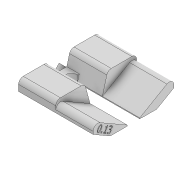
# Autodesk Inventor part: alex_clip
Saved by Autodesk Inventor 2022 (Build 260153000, 153)
## iProperties
Created: 2022-08-18
Part Number: alex_clip
Material: Generic
Document SubType Name: Modeling
Designer: dsdan
Density: 1 g/cm^3
Appearance: Default
Author: dsdan
Autodesk Inventor part; units mm, degrees
ref_plane "YZ Plane" through (0, 0, 0) normal (1, 0, 0) x (0, 1, 0)
ref_plane "XZ Plane" through (0, 0, 0) normal (0, 1, 0) x (-1, 0, 0)
ref_plane "XY Plane" through (0, 0, 0) normal (0, 0, 1) x (1, 0, 0)
sketch "Sketch1" plane through (0, 0, 0) normal (1, 0, 0) x (0, 1, 0)
  arc A0 (3.8, 2.5025) -> (-1, 4.4387) centre (0, 0) ccw
  line L0 (3.8, 2.5025) -> (3.8, -2.5025)
  line L1 (-1, 4.4387) -> (-1, -4.4387)
  arc A1 (3.8, -2.5025) -> (3.8, 2.5025) centre (0, 0) ccw construction
  arc A2 (-1, 4.4387) -> (-1, -4.4387) centre (0, 0) ccw construction
  arc A3 (-1, -4.4387) -> (3.8, -2.5025) centre (0, 0) ccw
  dimension "d0" = 9.1
  dimension "d5" = 4.8
  dimension "d40" = 3.8
  constraints: 9 point on circle, 4 centre point, 4 end point, 1 coincident, 1 vertical
  measures "d0" diameter of A0
  measures "d5" distance between parallel lines of L1 L0
  measures "d40" distance from line of point (0, 0) L0
extrude "Extrusion1" add sketch "Sketch1" along normal blind 28
sketch "Sketch9" plane through (28, 0, 0) normal (1, 0, 0) x (0, 0, -1)
  arc A0 (-2.5025, 3.8) -> (-4.4387, -1) centre (0, 0) ccw projected
  line L0 (-4.1788, 1.8) -> (4.1788, 1.8)
  arc A1 (4.4387, -1) -> (2.5025, 3.8) centre (0, 0) ccw projected
  line L1 (2.5025, 3.8) -> (-2.5025, 3.8) projected
  line L2 (-4.2305, 1.675) -> (4.2305, 1.675) construction
  dimension "d69" = 2.125
  dimension "d70" = 0.125
  constraints: 4 end point, 4 point on circle, 2 horizontal
  measures "d69" distance between parallel lines of L2 L1
  measures "d70" distance between parallel lines of L2 L0
extrude "Extrusion9" cut sketch "Sketch9" against normal blind 24
sketch "Sketch3" plane through (0, 3.8, 2.5025) normal (0, 1, 0) x (1, 0, 0)
  circle A0 centre (8, 2.5025) radius 2
  line L0 (8, 4.5025) -> (28, 4.5025)
  line L1 (8, 0.5025) -> (28, 0.5025)
  line L2 (28, 5.005) -> (28, 0) projected
  line L3 (0, 5.005) -> (0, 0) projected
  point P0 (0, 2.5025)
  dimension "d10" = 4
  dimension "d61" = 8
  constraints: 4 end point, 2 horizontal, 2 point on circle, 2 point on line, 2 tangent, 1 centre point, 1 horizontal alignment
  measures "d10" diameter of A0
  measures "d61" distance from line of L3 A0.centre
extrude "Extrusion3" cut sketch "Sketch3" against normal through all
sketch "Sketch6" plane through (28, 0, 0) normal (1, 0, 0) x (0, 0, -1)
  line L0 (-2, 1.8) -> (-2, -1) projected
  circle A0 centre (0, 0) radius 3.05
  line L1 (-2.6268, 1.55) -> (2.6268, 1.55)
  line L2 (-2.6268, -1.55) -> (2.6268, -1.55)
  dimension "d42" = 6.1
  dimension "d43" = 3.1
  dimension "d44" = 1.55
  constraints: 4 end point, 4 point on circle, 1 centre point, 1 coincident, 1 horizontal
  measures "d42" diameter of A0
  measures "d43" distance between parallel lines of L1 L2
  measures "d44" distance from line of point (0, 0) L1
extrude "Extrusion7" cut sketch "Sketch6" against normal through all contours A0 L2 L1
fillet "Fillet3" radius 0.3 2 edges at (14, 1.55, 2.6268) (14, 1.55, -2.6268)
sketch "Sketch7" plane through (8, 3.8, -2) normal (0, 0, 1) x (1, 0, 0)
  circle A0 centre (1, -3.8) radius 1.5
  line L0 (1, -5.3) -> (20, -5.3)
  line L1 (20, -5.3) -> (20, -2.3)
  line L2 (1, -2.3) -> (20, -2.3)
  line L3 (20, -4.8) -> (0, -4.8) projected
  line L4 (20, -2) -> (20, -2.25) projected
  line L5 (-8, -4.8) -> (-8, 0) projected
  dimension "d28" = 3
  dimension "d33" = 2.5
  dimension "d60" = 9
  constraints: 6 end point, 2 perpendicular, 2 point on circle, 2 tangent, 1 centre point, 1 collinear, 1 horizontal
  measures "d28" diameter of A0
  measures "d33" distance between parallel lines of L3 L2
  measures "d60" distance from line of L5 A0.centre
extrude "Extrusion6" cut sketch "Sketch7" along normal through all both and the other way through all
sketch "Sketch12" plane through (0, 0, 0) normal (-1, 0, 0) x (0, 0, 1)
  line L0 (-4.55, -1) -> (4.55, -1) construction
  line L1 (4.55, -1) -> (4.55, 2.5)
  line L2 (4.55, 2.5) -> (-4.55, 2.5) construction
  line L3 (-4.55, 2.5) -> (-4.55, -1)
  arc A0 (-2.5025, 3.8) -> (-4.4387, -1) centre (0, 0) ccw projected
  arc A1 (4.4387, -1) -> (2.5025, 3.8) centre (0, 0) ccw projected
  line L4 (-2.8814, -1) -> (-4.4387, -1) projected
  line L5 (-4.55, 2.5) -> (-2.05, 0)
  line L6 (-4.55, 2.5) -> (-1.0145, 2.5) construction
  line L7 (-2.05, 0) -> (2.05, 0)
  line L8 (2.05, 0) -> (4.55, 2.5)
  line L9 (-4.55, 2.5) -> (-4.55, 4.4728)
  line L10 (-4.55, 4.4728) -> (4.55, 4.4728)
  line L11 (4.55, 4.4728) -> (4.55, 2.5)
  dimension "d57" = 3.5
  dimension "d58" = 45
  dimension "d59" = 45
  constraints: 22 end point, 3 horizontal, 3 perpendicular, 2 parallel, 2 tangent, 1 collinear, 1 equal length, 1 vertical
  measures "d57" distance between parallel lines of L0 L2
  measures "d58" angle of L5 L6
  measures "d59" angle of L2 L8
extrude "Extrusion11" cut sketch "Sketch12" against normal blind 4 contours L8 L7 L5 L9 L10 L11
sketch "Sketch4" plane through (28, 0, 0) normal (1, 0, 0) x (0, 0, -1)
  arc A0 (-4.1788, 1.8) -> (-4.2956, 1.5) centre (0, 0) ccw projected
  line L0 (-2, 1.8) -> (-13, 8.1509)
  line L1 (-2, 1.8) -> (10.7017, 1.8) construction
  line L2 (-13, 8.1509) -> (-13, 1.5)
  line L3 (2.6153, 1.5) -> (4.2956, 1.5) projected
  line L4 (-4.2956, 1.5) -> (4.2956, 1.5) projected
  line L5 (-13, 1.5) -> (-4.2956, 1.5)
  arc A1 (4.2956, 1.5) -> (4.1788, 1.8) centre (0, 0) ccw projected
  line L6 (2, 1.8) -> (2, 1.55) projected
  line L7 (-4.2956, 1.5) -> (-2.6153, 1.5) projected
  line L8 (-2.4495, 1.55) -> (-2, 1.55) projected
  arc A2 (2.6153, 1.5) -> (2.4495, 1.55) centre (2.4495, 1.25) ccw projected
  line L9 (4.1788, 1.8) -> (2, 1.8) projected
  arc A3 (-2.4495, 1.55) -> (-2.6153, 1.5) centre (-2.4495, 1.25) ccw projected
  line L10 (-2, 1.55) -> (-2, 1.8) projected
  line L11 (-2, 1.8) -> (-4.1788, 1.8) projected
  line L12 (2, 1.55) -> (2.4495, 1.55) projected
  point P0 (-4.4387, -1)
  point P1 (-1.5, 2.3)
  dimension "d16" = 30
  dimension "d21" = 11
  constraints: 8 end point, 1 collinear, 1 equal length, 1 horizontal, 1 perpendicular
  measures "d16" angle of L1 L0
  measures "d21" distance from line of L0.start L2
extrude "Extrusion4" add sketch "Sketch4" against normal blind 12 contours A0 L5 L2 L0 L11
sketch "Sketch5" plane through (16, 0, 0) normal (-1, 0, 0) x (0, 0, 1)
  line L0 (-2, 1.8) -> (-2, 1.55) projected
  arc A0 (-4.1788, 1.8) -> (-4.2956, 1.5) centre (0, 0) ccw projected
  line L1 (-2, 1.8) -> (-3.7017, 8.1509)
  line L2 (-3.7017, 8.1509) -> (-13, 8.1509)
  line L3 (-13, 8.1509) -> (-13, 1.5)
  line L4 (13, 1.5) -> (2.6153, 1.5) projected
  arc A1 (-4.1788, 1.8) -> (-4.2956, 1.5) centre (0, 0) ccw projected
  line L5 (-13, 1.5) -> (-4.2956, 1.5)
  line L6 (-2.6153, 1.5) -> (-4.2956, 1.5) projected
  line L7 (-2, 1.55) -> (-2.4495, 1.55) projected
  arc A2 (-2.4495, 1.55) -> (-2.6153, 1.5) centre (-2.4495, 1.25) ccw projected
  line L8 (-4.1788, 1.8) -> (-2, 1.8) projected
  arc A3 (2.6153, 1.5) -> (2.4495, 1.55) centre (2.4495, 1.25) ccw projected
  line L9 (2.4495, 1.55) -> (2, 1.55) projected
  line L10 (2, 1.55) -> (2, 1.8) projected
  line L11 (2, 1.8) -> (13, 8.1509) projected
  line L12 (13, 8.1509) -> (13, 1.5) projected
  dimension "d25" = 11
  dimension "d49" = 75
  constraints: 8 end point, 2 horizontal, 1 perpendicular, 1 point on line
  measures "d25" distance between parallel lines of L3 L0
  measures "d49" angle of L8 L1
extrude "Extrusion5" add sketch "Sketch5" along normal blind 12 contours L8 A0 L5 L3 L2 L1
fillet "Fillet1" radius 1.5 3 edges at (22, 8.1509, 13) (10, 8.1509, -13) (10, 8.1509, -3.7017)
mirror "Mirror1" about plane through (0, 0, 0) normal (0, 0, 1) of "Extrusion5", "Extrusion4", "Fillet1"
sketch "Sketch8" plane through (28, 0, 0) normal (1, 0, 0) x (0, 0, -1)
  line L0 (13, 1.5) -> (2.6153, 1.5) projected
  line L1 (-2.6153, 1.5) -> (-4.2956, 1.5) projected
  line L2 (-13, 5.5528) -> (-13, 1.5) projected
  line L3 (-2, 1.8) -> (-10.75, 6.8518) construction
  line L4 (2, 1.8) -> (2, 1.55) projected
  line L5 (2, 1.55) -> (2.4495, 1.55) projected
  arc A0 (2.6153, 1.5) -> (2.4495, 1.55) centre (2.4495, 1.25) ccw projected
  line L6 (-13, 1.5) -> (-2.6153, 1.5) projected
  arc A1 (-10.75, 6.8518) -> (-13, 5.5528) centre (-11.5, 5.5528) ccw projected
  line L7 (-13, 4.6868) -> (-7.4804, 1.5)
  arc A2 (-2.4495, 1.55) -> (-2.6153, 1.5) centre (-2.4495, 1.25) ccw projected
  line L8 (-2.4495, 1.55) -> (-2, 1.55) projected
  line L9 (-2, 1.55) -> (-2, 1.8) projected
  line L10 (13, 5.5528) -> (13, 1.5) projected
  arc A3 (13, 5.5528) -> (10.75, 6.8518) centre (11.5, 5.5528) ccw projected
  line L11 (2, 1.8) -> (10.75, 6.8518) projected
  arc A4 (-10.75, 6.8518) -> (-13, 5.5528) centre (-11.5, 5.5528) ccw projected
  line L12 (-13, 5.5528) -> (-13, 1.5) projected
  line L13 (-2, 1.8) -> (-10.75, 6.8518) construction
  point P0 (0, 0)
  point P1 (-10.5, 7.4962)
  point P2 (-13, 4.6868)
  dimension "d68" = 3
  constraints: 2 end point, 1 parallel, 1 point on line, 1 other
  measures "d68" distance between parallel lines of L3 L7
extrude "Extrusion8" cut sketch "Sketch8" against normal through all contours L7 L6 L2
mirror "Mirror2" about plane through (0, 0, 0) normal (0, 0, 1) of "Extrusion8"
sketch "Sketch11" plane through (0, 3.8, 2.5025) normal (0, 1, 0) x (1, 0, 0)
  arc A0 (8, 4.5025) -> (8, 0.5025) centre (8, 2.5025) ccw projected
  arc A1 (8, 4.5025) -> (8, 0.5025) centre (8, 2.5025) ccw projected
  line L0 (4, 0.5025) -> (4, -0.4975)
  line L1 (4, -0.4975) -> (8, -0.4975)
  line L2 (8, -0.4975) -> (8, 0.5025)
  line L3 (8, 4.5025) -> (4, 4.5025) construction
  line L4 (4, 4.5025) -> (4, 5.5025)
  line L5 (4, 5.5025) -> (8, 5.5025)
  line L6 (8, 5.5025) -> (8, 4.5025)
  line L7 (4, 4.5025) -> (4, 0.5025) projected
  line L8 (8, 4.5025) -> (4, 4.5025) projected
  line L9 (4, 0.5025) -> (8, 0.5025) construction
  point P0 (7.5077, 4.441)
  constraints: 12 end point, 2 collinear, 2 parallel
extrude "Extrusion10" add sketch "Sketch11" against normal up to surface (2 mm away)
sketch "Sketch13" plane through (4, 1.6589, -7.7555) normal (0, -0.8660254, -0.5) x (0, 0.5, -0.8660254)
  line L0 (-0.3177, 24) -> (6.0558, 24) construction
  line L1 (6.0558, 24) -> (6.0558, 12) construction
  line L2 (6.0558, 12) -> (-0.3177, 12) construction
  line L3 (-0.3177, 12) -> (-0.3177, 24) construction
  line L4 (6.0558, 24) -> (6.0558, 0) projected
  line L5 (-0.3177, 12) -> (6.0558, 12) construction
  line L6 (6.0558, 12) -> (6.0558, 0) construction
  line L7 (6.0558, 0) -> (-0.3177, 0) construction
  line L8 (-0.3177, 0) -> (-0.3177, 12) construction
  line L9 (-0.3177, 0) -> (-0.3177, 24) projected
  line L10 (7.0378, 12) -> (6.4888, 12) projected
  line L11 (7.0378, 0) -> (6.0558, 0) projected
  line L12 (-0.3177, 24) -> (6.0558, 24) projected
  spline S0 degree 2 poles (1.0114, 21.0934) (0.9187, 21.0934) (0.7355, 21.0482) (0.647, 21.0132) knots 0 0 0 1 2 2 2
  spline S1 degree 2 poles (0.647, 21.0132) (0.5647, 20.9782) (0.4433, 20.9041) (0.3959, 20.8711) knots 0 0 0 1 2 2 2
  line L13 (0.3959, 20.8711) -> (0.3753, 20.8711)
  line L14 (0.3753, 20.8711) -> (0.3753, 21.2313)
  spline S2 degree 2 poles (0.3753, 21.2313) (0.4865, 21.291) (0.8673, 21.3878) (1.0381, 21.3878) knots 0 0 0 1 2 2 2
  spline S3 degree 2 poles (1.0381, 21.3878) (1.211, 21.3878) (1.4683, 21.3178) (1.5733, 21.2437) knots 0 0 0 1 2 2 2
  spline S4 degree 2 poles (1.5733, 21.2437) (1.6844, 21.1634) (1.7997, 20.9308) (1.7997, 20.7744) knots 0 0 0 1 2 2 2
  spline S5 degree 2 poles (1.7997, 20.7744) (1.7997, 20.5644) (1.5239, 20.2475) (1.3304, 20.2063) knots 0 0 0 1 2 2 2
  line L15 (1.3304, 20.2063) -> (1.3304, 20.1816)
  spline S6 degree 2 poles (1.3304, 20.1816) (1.4107, 20.1651) (1.5939, 20.091) (1.6721, 20.0169) knots 0 0 0 1 2 2 2
  spline S7 degree 2 poles (1.6721, 20.0169) (1.7503, 19.9449) (1.8491, 19.7143) (1.8491, 19.5476) knots 0 0 0 1 2 2 2
  spline S8 degree 2 poles (1.8491, 19.5476) (1.8491, 19.3768) (1.7318, 19.0865) (1.6247, 18.9754) knots 0 0 0 1 2 2 2
  spline S9 degree 2 poles (1.6247, 18.9754) (1.5136, 18.8601) (1.1987, 18.7407) (0.999, 18.7407) knots 0 0 0 1 2 2 2
  spline S10 degree 2 poles (0.999, 18.7407) (0.8076, 18.7407) (0.433, 18.8334) (0.3053, 18.8972) knots 0 0 0 1 2 2 2
  line L16 (0.3053, 18.8972) -> (0.3053, 19.2574)
  line L17 (0.3053, 19.2574) -> (0.33, 19.2574)
  spline S11 degree 2 poles (0.33, 19.2574) (0.4371, 19.1792) (0.7994, 19.0351) (0.9784, 19.0351) knots 0 0 0 1 2 2 2
  spline S12 degree 2 poles (0.9784, 19.0351) (1.0834, 19.0351) (1.2934, 19.101) (1.3633, 19.1771) knots 0 0 0 1 2 2 2
  spline S13 degree 2 poles (1.3633, 19.1771) (1.4313, 19.2533) (1.5033, 19.4344) (1.5033, 19.5723) knots 0 0 0 1 2 2 2
  spline S14 degree 2 poles (1.5033, 19.5723) (1.5033, 19.7102) (1.423, 19.8893) (1.351, 19.9408) knots 0 0 0 1 2 2 2
  spline S15 degree 2 poles (1.351, 19.9408) (1.2789, 19.9922) (1.0834, 20.0313) (0.9681, 20.0313) knots 0 0 0 1 2 2 2
  line L18 (0.9681, 20.0313) -> (0.8241, 20.0313)
  line L19 (0.8241, 20.0313) -> (0.8241, 20.3133)
  line L20 (0.8241, 20.3133) -> (0.9373, 20.3133)
  spline S16 degree 2 poles (0.9373, 20.3133) (1.1657, 20.3133) (1.4539, 20.5315) (1.4539, 20.7394) knots 0 0 0 1 2 2 2
  spline S17 degree 2 poles (1.4539, 20.7394) (1.4539, 20.8361) (1.3798, 20.9741) (1.3201, 21.0152) knots 0 0 0 1 2 2 2
  spline S18 degree 2 poles (1.3201, 21.0152) (1.2563, 21.0584) (1.0999, 21.0934) (1.0114, 21.0934) knots 0 0 0 1 2 2 2
  spline S19 degree 2 poles (3.8128, 20.0643) (3.8128, 19.3809) (3.4155, 18.7407) (3.0018, 18.7407) knots 0 0 0 1 2 2 2
  spline S20 degree 2 poles (3.0018, 18.7407) (2.5819, 18.7407) (2.1887, 19.3932) (2.1887, 20.0622) knots 0 0 0 1 2 2 2
  spline S21 degree 2 poles (2.1887, 20.0622) (2.1887, 20.7497) (2.586, 21.3857) (3.0018, 21.3857) knots 0 0 0 1 2 2 2
  spline S22 degree 2 poles (3.0018, 21.3857) (3.4196, 21.3857) (3.8128, 20.7271) (3.8128, 20.0643) knots 0 0 0 1 2 2 2
  spline S23 degree 2 poles (3.3764, 19.2903) (3.4258, 19.4159) (3.467, 19.8029) (3.467, 20.0643) knots 0 0 0 1 2 2 2
  spline S24 degree 2 poles (3.467, 20.0643) (3.467, 20.3257) (3.4258, 20.7106) (3.3743, 20.8403) knots 0 0 0 1 2 2 2
  spline S25 degree 2 poles (3.3743, 20.8403) (3.3229, 20.9699) (3.1438, 21.1037) (3.0018, 21.1037) knots 0 0 0 1 2 2 2
  spline S26 degree 2 poles (3.0018, 21.1037) (2.8598, 21.1037) (2.6766, 20.9699) (2.623, 20.8361) knots 0 0 0 1 2 2 2
  spline S27 degree 2 poles (2.623, 20.8361) (2.5716, 20.7065) (2.5345, 20.3113) (2.5345, 20.0622) knots 0 0 0 1 2 2 2
  spline S28 degree 2 poles (2.5345, 20.0622) (2.5345, 19.7946) (2.5675, 19.4365) (2.621, 19.2965) knots 0 0 0 1 2 2 2
  spline S29 degree 2 poles (2.621, 19.2965) (2.6704, 19.1648) (2.8536, 19.0227) (3.0018, 19.0227) knots 0 0 0 1 2 2 2
  spline S30 degree 2 poles (3.0018, 19.0227) (3.1418, 19.0227) (3.3249, 19.1565) (3.3764, 19.2903) knots 0 0 0 1 2 2 2
  spline S31 degree 2 poles (5.4245, 20.7291) (5.4245, 20.4553) (5.0498, 20.0807) (4.7761, 20.0807) knots 0 0 0 1 2 2 2
  spline S32 degree 2 poles (4.7761, 20.0807) (4.5044, 20.0807) (4.1256, 20.4533) (4.1256, 20.7291) knots 0 0 0 1 2 2 2
  spline S33 degree 2 poles (4.1256, 20.7291) (4.1256, 21.0029) (4.5003, 21.3775) (4.7761, 21.3775) knots 0 0 0 1 2 2 2
  spline S34 degree 2 poles (4.7761, 21.3775) (5.0498, 21.3775) (5.4245, 21.0029) (5.4245, 20.7291) knots 0 0 0 1 2 2 2
  spline S35 degree 2 poles (5.1569, 20.7291) (5.1569, 20.8938) (4.9387, 21.1181) (4.7761, 21.1181) knots 0 0 0 1 2 2 2
  spline S36 degree 2 poles (4.7761, 21.1181) (4.6114, 21.1181) (4.3932, 20.8938) (4.3932, 20.7291) knots 0 0 0 1 2 2 2
  spline S37 degree 2 poles (4.3932, 20.7291) (4.3932, 20.5624) (4.6155, 20.3401) (4.7761, 20.3401) knots 0 0 0 1 2 2 2
  spline S38 degree 2 poles (4.7761, 20.3401) (4.9387, 20.3401) (5.1569, 20.5665) (5.1569, 20.7291) knots 0 0 0 1 2 2 2
  line L21 (2.587, 14.6122) -> (1.3479, 14.6122)
  line L22 (1.3479, 14.6122) -> (1.3479, 14.8716)
  line L23 (1.3479, 14.8716) -> (1.809, 14.8716)
  line L24 (1.809, 14.8716) -> (1.809, 16.5738)
  line L25 (1.809, 16.5738) -> (1.3479, 16.5738)
  line L26 (1.3479, 16.5738) -> (1.3479, 16.8064)
  spline S39 degree 2 poles (1.3479, 16.8064) (1.6093, 16.8064) (1.8563, 16.9546) (1.8728, 17.1605) knots 0 0 0 1 2 2 2
  line L27 (1.8728, 17.1605) -> (2.1362, 17.1605)
  line L28 (2.1362, 17.1605) -> (2.1362, 14.8716)
  line L29 (2.1362, 14.8716) -> (2.587, 14.8716)
  line L30 (2.587, 14.8716) -> (2.587, 14.6122)
  line L31 (4.6207, 14.6122) -> (3.0543, 14.6122)
  line L32 (3.0543, 14.6122) -> (3.0543, 14.9724)
  spline S40 degree 2 poles (3.0543, 14.9724) (3.2231, 15.1309) (3.5236, 15.4253) (3.6677, 15.5838) knots 0 0 0 1 2 2 2
  spline S41 degree 2 poles (3.6677, 15.5838) (3.9579, 15.9028) (4.1699, 16.2857) (4.1699, 16.4894) knots 0 0 0 1 2 2 2
  spline S42 degree 2 poles (4.1699, 16.4894) (4.1699, 16.5965) (4.104, 16.757) (4.0443, 16.8085) knots 0 0 0 1 2 2 2
  spline S43 degree 2 poles (4.0443, 16.8085) (3.9846, 16.8599) (3.8282, 16.9114) (3.7335, 16.9114) knots 0 0 0 1 2 2 2
  spline S44 degree 2 poles (3.7335, 16.9114) (3.643, 16.9114) (3.4577, 16.8661) (3.3733, 16.8311) knots 0 0 0 1 2 2 2
  spline S45 degree 2 poles (3.3733, 16.8311) (3.3013, 16.8023) (3.1675, 16.72) (3.1263, 16.6912) knots 0 0 0 1 2 2 2
  line L33 (3.1263, 16.6912) -> (3.1078, 16.6912)
  line L34 (3.1078, 16.6912) -> (3.1078, 17.0534)
  spline S46 degree 2 poles (3.1078, 17.0534) (3.2128, 17.1049) (3.5894, 17.2057) (3.7582, 17.2057) knots 0 0 0 1 2 2 2
  spline S47 degree 2 poles (3.7582, 17.2057) (4.1143, 17.2057) (4.5157, 16.8291) (4.5157, 16.508) knots 0 0 0 1 2 2 2
  spline S48 degree 2 poles (4.5157, 16.508) (4.5157, 16.3577) (4.4457, 16.1066) (4.384, 15.9995) knots 0 0 0 1 2 2 2
  spline S49 degree 2 poles (4.384, 15.9995) (4.3222, 15.8884) (4.1431, 15.6702) (4.0443, 15.5652) knots 0 0 0 1 2 2 2
  spline S50 degree 2 poles (4.0443, 15.5652) (3.8838, 15.3903) (3.4906, 15.0157) (3.3733, 14.9066) knots 0 0 0 1 2 2 2
  line L35 (3.3733, 14.9066) -> (4.6207, 14.9066)
  line L36 (4.6207, 14.9066) -> (4.6207, 14.6122)
  line L37 (1.9212, 8.9586) -> (0.822, 6.7994)
  line L38 (0.822, 6.7994) -> (0.4597, 6.7994)
  line L39 (0.4597, 6.7994) -> (1.6206, 9.0409)
  line L40 (1.6206, 9.0409) -> (0.3095, 9.0409)
  line L41 (0.3095, 9.0409) -> (0.3095, 9.3394)
  line L42 (0.3095, 9.3394) -> (1.9212, 9.3394)
  line L43 (1.9212, 9.3394) -> (1.9212, 8.9586)
  spline S51 degree 2 poles (3.7716, 7.6063) (3.7716, 7.4231) (3.6543, 7.1102) (3.5472, 6.995) knots 0 0 0 1 2 2 2
  spline S52 degree 2 poles (3.5472, 6.995) (3.4402, 6.8797) (3.1212, 6.7459) (2.9236, 6.7459) knots 0 0 0 1 2 2 2
  spline S53 degree 2 poles (2.9236, 6.7459) (2.7424, 6.7459) (2.3884, 6.8262) (2.2587, 6.89) knots 0 0 0 1 2 2 2
  line L44 (2.2587, 6.89) -> (2.2587, 7.2502)
  line L45 (2.2587, 7.2502) -> (2.2834, 7.2502)
  spline S54 degree 2 poles (2.2834, 7.2502) (2.3225, 7.2214) (2.4687, 7.1473) (2.5572, 7.1143) knots 0 0 0 1 2 2 2
  spline S55 degree 2 poles (2.5572, 7.1143) (2.658, 7.0793) (2.8248, 7.0402) (2.9297, 7.0402) knots 0 0 0 1 2 2 2
  spline S56 degree 2 poles (2.9297, 7.0402) (3.0327, 7.0402) (3.2261, 7.1143) (3.2961, 7.1946) knots 0 0 0 1 2 2 2
  spline S57 degree 2 poles (3.2961, 7.1946) (3.3599, 7.2708) (3.4258, 7.4725) (3.4258, 7.6083) knots 0 0 0 1 2 2 2
  spline S58 degree 2 poles (3.4258, 7.6083) (3.4258, 7.7442) (3.3517, 7.9171) (3.2817, 7.9747) knots 0 0 0 1 2 2 2
  spline S59 degree 2 poles (3.2817, 7.9747) (3.2097, 8.0385) (2.9956, 8.0921) (2.8659, 8.0921) knots 0 0 0 1 2 2 2
  spline S60 degree 2 poles (2.8659, 8.0921) (2.726, 8.0921) (2.4481, 8.0488) (2.3637, 8.0303) knots 0 0 0 1 2 2 2
  line L46 (2.3637, 8.0303) -> (2.3637, 9.3394)
  line L47 (2.3637, 9.3394) -> (3.7572, 9.3394)
  line L48 (3.7572, 9.3394) -> (3.7572, 9.0409)
  line L49 (3.7572, 9.0409) -> (2.691, 9.0409)
  line L50 (2.691, 9.0409) -> (2.691, 8.3638)
  spline S61 degree 2 poles (2.691, 8.3638) (2.7527, 8.372) (2.8721, 8.3782) (2.9215, 8.3782) knots 0 0 0 1 2 2 2
  spline S62 degree 2 poles (2.9215, 8.3782) (3.1171, 8.3782) (3.3867, 8.3144) (3.5102, 8.2197) knots 0 0 0 1 2 2 2
  spline S63 degree 2 poles (3.5102, 8.2197) (3.6358, 8.125) (3.7716, 7.8368) (3.7716, 7.6063) knots 0 0 0 1 2 2 2
  spline S64 degree 2 poles (5.4245, 8.7343) (5.4245, 8.4605) (5.0498, 8.0859) (4.7761, 8.0859) knots 0 0 0 1 2 2 2
  spline S65 degree 2 poles (4.7761, 8.0859) (4.5044, 8.0859) (4.1256, 8.4584) (4.1256, 8.7343) knots 0 0 0 1 2 2 2
  spline S66 degree 2 poles (4.1256, 8.7343) (4.1256, 9.008) (4.5003, 9.3826) (4.7761, 9.3826) knots 0 0 0 1 2 2 2
  spline S67 degree 2 poles (4.7761, 9.3826) (5.0498, 9.3826) (5.4245, 9.008) (5.4245, 8.7343) knots 0 0 0 1 2 2 2
  spline S68 degree 2 poles (5.1569, 8.7343) (5.1569, 8.8989) (4.9387, 9.1233) (4.7761, 9.1233) knots 0 0 0 1 2 2 2
  spline S69 degree 2 poles (4.7761, 9.1233) (4.6114, 9.1233) (4.3932, 8.8989) (4.3932, 8.7343) knots 0 0 0 1 2 2 2
  spline S70 degree 2 poles (4.3932, 8.7343) (4.3932, 8.5675) (4.6155, 8.3452) (4.7761, 8.3452) knots 0 0 0 1 2 2 2
  spline S71 degree 2 poles (4.7761, 8.3452) (4.9387, 8.3452) (5.1569, 8.5716) (5.1569, 8.7343) knots 0 0 0 1 2 2 2
  line L51 (2.587, 2.6174) -> (1.3479, 2.6174)
  line L52 (1.3479, 2.6174) -> (1.3479, 2.8767)
  line L53 (1.3479, 2.8767) -> (1.809, 2.8767)
  line L54 (1.809, 2.8767) -> (1.809, 4.579)
  line L55 (1.809, 4.579) -> (1.3479, 4.579)
  line L56 (1.3479, 4.579) -> (1.3479, 4.8116)
  spline S72 degree 2 poles (1.3479, 4.8116) (1.6093, 4.8116) (1.8563, 4.9598) (1.8728, 5.1656) knots 0 0 0 1 2 2 2
  line L57 (1.8728, 5.1656) -> (2.1362, 5.1656)
  line L58 (2.1362, 5.1656) -> (2.1362, 2.8767)
  line L59 (2.1362, 2.8767) -> (2.587, 2.8767)
  line L60 (2.587, 2.8767) -> (2.587, 2.6174)
  line L61 (4.6207, 2.6174) -> (3.0543, 2.6174)
  line L62 (3.0543, 2.6174) -> (3.0543, 2.9776)
  spline S73 degree 2 poles (3.0543, 2.9776) (3.2231, 3.1361) (3.5236, 3.4304) (3.6677, 3.5889) knots 0 0 0 1 2 2 2
  spline S74 degree 2 poles (3.6677, 3.5889) (3.9579, 3.9079) (4.1699, 4.2908) (4.1699, 4.4946) knots 0 0 0 1 2 2 2
  spline S75 degree 2 poles (4.1699, 4.4946) (4.1699, 4.6016) (4.104, 4.7622) (4.0443, 4.8136) knots 0 0 0 1 2 2 2
  spline S76 degree 2 poles (4.0443, 4.8136) (3.9846, 4.8651) (3.8282, 4.9165) (3.7335, 4.9165) knots 0 0 0 1 2 2 2
  spline S77 degree 2 poles (3.7335, 4.9165) (3.643, 4.9165) (3.4577, 4.8713) (3.3733, 4.8363) knots 0 0 0 1 2 2 2
  spline S78 degree 2 poles (3.3733, 4.8363) (3.3013, 4.8074) (3.1675, 4.7251) (3.1263, 4.6963) knots 0 0 0 1 2 2 2
  line L63 (3.1263, 4.6963) -> (3.1078, 4.6963)
  line L64 (3.1078, 4.6963) -> (3.1078, 5.0586)
  spline S79 degree 2 poles (3.1078, 5.0586) (3.2128, 5.11) (3.5894, 5.2109) (3.7582, 5.2109) knots 0 0 0 1 2 2 2
  spline S80 degree 2 poles (3.7582, 5.2109) (4.1143, 5.2109) (4.5157, 4.8342) (4.5157, 4.5131) knots 0 0 0 1 2 2 2
  spline S81 degree 2 poles (4.5157, 4.5131) (4.5157, 4.3628) (4.4457, 4.1117) (4.384, 4.0047) knots 0 0 0 1 2 2 2
  spline S82 degree 2 poles (4.384, 4.0047) (4.3222, 3.8935) (4.1431, 3.6754) (4.0443, 3.5704) knots 0 0 0 1 2 2 2
  spline S83 degree 2 poles (4.0443, 3.5704) (3.8838, 3.3954) (3.4906, 3.0208) (3.3733, 2.9117) knots 0 0 0 1 2 2 2
  line L65 (3.3733, 2.9117) -> (4.6207, 2.9117)
  line L66 (4.6207, 2.9117) -> (4.6207, 2.6174)
  point P0 (-7.5459, -4)
  dimension "forewing_angle" = 30
  dimension "hindwing_angle" = 75
  dimension "forewingbase_width" = 12
  dimension "hindwingbase_width" = 12
  constraints: 8 collinear, 4 other
extrude "Extrusion12" cut sketch "Sketch13" against normal blind 0.75
sketch "Sketch15" plane through (28, 0, 0) normal (1, 0, 0) x (0, 0, -1)
  line L0 (-11.5, 7.2848) -> (-5.539, 3.8432) construction
  line L1 (-5.539, 3.8432) -> (-7.039, 1.2452) construction
  line L2 (-7.039, 1.2452) -> (-13, 4.6868) construction
  line L3 (-13, 4.6868) -> (-11.5, 7.2848) construction
  line L4 (-2, 1.8) -> (-10.75, 6.8518) projected
  spline S0 degree 2 poles (-10.3755, 4.9036) (-10.6446, 4.4376) (-11.1675, 4.1575) (-11.4496, 4.3203) knots 0 0 0 1 2 2 2
  spline S1 degree 2 poles (-11.4496, 4.3203) (-11.736, 4.4857) (-11.7472, 5.0854) (-11.4838, 5.5415) knots 0 0 0 1 2 2 2
  spline S2 degree 2 poles (-11.4838, 5.5415) (-11.2131, 6.0104) (-10.6918, 6.2877) (-10.4083, 6.124) knots 0 0 0 1 2 2 2
  spline S3 degree 2 poles (-10.4083, 6.124) (-10.1234, 5.9595) (-10.1146, 5.3555) (-10.3755, 4.9036) knots 0 0 0 1 2 2 2
  spline S4 degree 2 poles (-10.9778, 4.5476) (-10.8947, 4.6138) (-10.7143, 4.8615) (-10.6113, 5.0397) knots 0 0 0 1 2 2 2
  spline S5 degree 2 poles (-10.6113, 5.0397) (-10.5084, 5.218) (-10.385, 5.4967) (-10.369, 5.6053) knots 0 0 0 1 2 2 2
  spline S6 degree 2 poles (-10.369, 5.6053) (-10.353, 5.714) (-10.4225, 5.8758) (-10.5193, 5.9317) knots 0 0 0 1 2 2 2
  spline S7 degree 2 poles (-10.5193, 5.9317) (-10.6162, 5.9876) (-10.7938, 5.9685) (-10.8829, 5.8983) knots 0 0 0 1 2 2 2
  spline S8 degree 2 poles (-10.8829, 5.8983) (-10.9691, 5.8301) (-11.1499, 5.5752) (-11.248, 5.4054) knots 0 0 0 1 2 2 2
  spline S9 degree 2 poles (-11.248, 5.4054) (-11.3533, 5.2229) (-11.4719, 4.9657) (-11.4905, 4.8492) knots 0 0 0 1 2 2 2
  spline S10 degree 2 poles (-11.4905, 4.8492) (-11.5087, 4.7399) (-11.4397, 4.571) (-11.3386, 4.5126) knots 0 0 0 1 2 2 2
  spline S11 degree 2 poles (-11.3386, 4.5126) (-11.2432, 4.4575) (-11.0656, 4.4766) (-10.9778, 4.5476) knots 0 0 0 1 2 2 2
  line L5 (-10.2818, 3.6948) -> (-10.5597, 3.8552)
  line L6 (-10.5597, 3.8552) -> (-10.3685, 4.1865)
  line L7 (-10.3685, 4.1865) -> (-10.0906, 4.026)
  line L8 (-10.0906, 4.026) -> (-10.2818, 3.6948)
  line L9 (-8.9512, 2.9265) -> (-9.7962, 3.4144)
  line L10 (-9.7962, 3.4144) -> (-9.6941, 3.5912)
  line L11 (-9.6941, 3.5912) -> (-9.3797, 3.4097)
  line L12 (-9.3797, 3.4097) -> (-8.7095, 4.5705)
  line L13 (-8.7095, 4.5705) -> (-9.0239, 4.752)
  line L14 (-9.0239, 4.752) -> (-8.9323, 4.9106)
  spline S12 degree 2 poles (-8.9323, 4.9106) (-8.7541, 4.8077) (-8.5273, 4.8115) (-8.435, 4.9454) knots 0 0 0 1 2 2 2
  line L15 (-8.435, 4.9454) -> (-8.2553, 4.8417)
  line L16 (-8.2553, 4.8417) -> (-9.1565, 3.2808)
  line L17 (-9.1565, 3.2808) -> (-8.8491, 3.1034)
  line L18 (-8.8491, 3.1034) -> (-8.9512, 2.9265)
  spline S13 degree 2 poles (-7.26, 4.0405) (-7.3232, 4.077) (-7.4659, 4.1183) (-7.54, 4.1292) knots 0 0 0 1 2 2 2
  spline S14 degree 2 poles (-7.54, 4.1292) (-7.61, 4.1378) (-7.7219, 4.1351) (-7.7672, 4.1313) knots 0 0 0 1 2 2 2
  line L19 (-7.7672, 4.1313) -> (-7.7812, 4.1394)
  line L20 (-7.7812, 4.1394) -> (-7.6394, 4.385)
  spline S15 degree 2 poles (-7.6394, 4.385) (-7.5401, 4.3819) (-7.2424, 4.298) (-7.1259, 4.2307) knots 0 0 0 1 2 2 2
  spline S16 degree 2 poles (-7.1259, 4.2307) (-7.008, 4.1627) (-6.8601, 4.0136) (-6.8176, 3.9218) knots 0 0 0 1 2 2 2
  spline S17 degree 2 poles (-6.8176, 3.9218) (-6.7735, 3.8233) (-6.7864, 3.6193) (-6.848, 3.5126) knots 0 0 0 1 2 2 2
  spline S18 degree 2 poles (-6.848, 3.5126) (-6.9307, 3.3694) (-7.2436, 3.2619) (-7.3917, 3.31) knots 0 0 0 1 2 2 2
  line L21 (-7.3917, 3.31) -> (-7.4014, 3.2931)
  spline S19 degree 2 poles (-7.4014, 3.2931) (-7.3532, 3.2503) (-7.2574, 3.1277) (-7.2333, 3.0463) knots 0 0 0 1 2 2 2
  spline S20 degree 2 poles (-7.2333, 3.0463) (-7.2083, 2.9664) (-7.2317, 2.7703) (-7.2973, 2.6566) knots 0 0 0 1 2 2 2
  spline S21 degree 2 poles (-7.2973, 2.6566) (-7.3646, 2.5401) (-7.5588, 2.3884) (-7.6756, 2.3547) knots 0 0 0 1 2 2 2
  spline S22 degree 2 poles (-7.6756, 2.3547) (-7.7968, 2.3199) (-8.0585, 2.3625) (-8.1947, 2.4411) knots 0 0 0 1 2 2 2
  spline S23 degree 2 poles (-8.1947, 2.4411) (-8.3252, 2.5164) (-8.5442, 2.7271) (-8.6061, 2.8209) knots 0 0 0 1 2 2 2
  line L22 (-8.6061, 2.8209) -> (-8.4643, 3.0665)
  line L23 (-8.4643, 3.0665) -> (-8.4474, 3.0568)
  spline S24 degree 2 poles (-8.4474, 3.0568) (-8.4052, 2.9613) (-8.2149, 2.7204) (-8.0928, 2.6499) knots 0 0 0 1 2 2 2
  spline S25 degree 2 poles (-8.0928, 2.6499) (-8.0212, 2.6086) (-7.8521, 2.5708) (-7.7744, 2.5952) knots 0 0 0 1 2 2 2
  spline S26 degree 2 poles (-7.7744, 2.5952) (-7.6981, 2.6204) (-7.5777, 2.7156) (-7.5234, 2.8096) knots 0 0 0 1 2 2 2
  spline S27 degree 2 poles (-7.5234, 2.8096) (-7.4691, 2.9036) (-7.4533, 3.0574) (-7.4822, 3.1208) knots 0 0 0 1 2 2 2
  spline S28 degree 2 poles (-7.4822, 3.1208) (-7.5111, 3.1843) (-7.629, 3.2879) (-7.7076, 3.3333) knots 0 0 0 1 2 2 2
  line L24 (-7.7076, 3.3333) -> (-7.8059, 3.39)
  line L25 (-7.8059, 3.39) -> (-7.6948, 3.5823)
  line L26 (-7.6948, 3.5823) -> (-7.6176, 3.5377)
  spline S29 degree 2 poles (-7.6176, 3.5377) (-7.4618, 3.4478) (-7.1794, 3.4831) (-7.0976, 3.6249) knots 0 0 0 1 2 2 2
  spline S30 degree 2 poles (-7.0976, 3.6249) (-7.0595, 3.6909) (-7.0557, 3.8141) (-7.0802, 3.8656) knots 0 0 0 1 2 2 2
  spline S31 degree 2 poles (-7.0802, 3.8656) (-7.1067, 3.9202) (-7.1996, 4.0057) (-7.26, 4.0405) knots 0 0 0 1 2 2 2
  point P0 (0, 0)
  dimension "wingbase_lift" = 0.125
  constraints: 1 coincident, 1 collinear, 2 other
extrude "Extrusion14" cut sketch "Sketch15" against normal blind 0.75
equation "\"d70\" = wingbase_lift"
equation "\"d47\" = 2 * forewingbase_width"
equation "\"d44\" = 0.5 * d43"
equation "\"d16\" = forewing_angle"
equation "\"d21\" = wingbase_length"
equation "\"d17\" = forewingbase_width"
equation "\"d25\" = wingbase_length"
equation "\"d49\" = hindwing_angle"
equation "\"d23\" = hindwingbase_width"
equation "\"forewing_angle\" = 30deg"
equation "\"hindwing_angle\" = 75deg"
equation "\"forewingbase_width\" = 12"
equation "\"hindwingbase_width\" = 12"
equation "\"wingbase_lift\" = 0.125"
equation "\"wingbase_length\" = 11"
body "Solid1"
